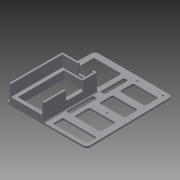
# Autodesk Inventor part: control pod layer a
Saved by Autodesk Inventor 2014 SP1 (Build 180222100, 222)
## iProperties
Created: 2017-06-28
Part Number: control pod layer a
Material: Generic
Document SubType Name: Modeling
Designer: kteo17
Density: 1 g/cm^3
Appearance: Default
Author: kteo17
Autodesk Inventor part; units mm, degrees
ref_plane "YZ Plane" through (0, 0, 0) normal (1, 0, 0) x (0, 1, 0)
ref_plane "XZ Plane" through (0, 0, 0) normal (0, 1, 0) x (-1, 0, 0)
ref_plane "XY Plane" through (0, 0, 0) normal (0, 0, 1) x (1, 0, 0)
sketch "Sketch1" plane through (0, 0, 0) normal (0, 0, 1) x (1, 0, 0)
  line L0 (3.175, 0) -> (146.685, 0)
  line L1 (0, 161.925) -> (149.86, 161.925)
  line L2 (0, 161.925) -> (3.175, 0)
  line L3 (149.86, 161.925) -> (146.685, 0)
  point P0 (0, 0)
  dimension "d60" = 143.51
  dimension "d62" = 161.925
  dimension "d63" = 149.86
  constraints: 8 end point, 1 horizontal
  measures "d60" distance of L0.start L0.end
  measures "d62" distance between parallel lines of L0 L1
  measures "d63" distance of L1.start L1.end
extrude "Extrusion1" add sketch "Sketch1" along normal blind 3.048
fillet "Fillet1" radius 6.35 4 edges at (146.685, 0, 1.524) (149.86, 161.925, 1.524) (0, 161.925, 1.524) (3.175, 0, 1.524)
sketch "Sketch3" plane through (0, 0, 3.048) normal (0, 0, 1) x (1, 0, 0)
  circle A0 centre (59.9281, 7.9375) radius 1.5875
  circle A1 centre (12.7, 7.9375) radius 1.5875
  circle A2 centre (36.3141, 87.9475) radius 1.5875
  point P0 (0, 0)
  dimension "d127" = 3.175
  dimension "d128" = 3.175
  dimension "d129" = 3.175
  dimension "d130" = 47.2281
  dimension "d131" = 80.01
  dimension "d132" = 23.6141
  constraints: 3 centre point
  measures "d127" diameter of A2
  measures "d128" diameter of A1
  measures "d129" diameter of A0
  measures "d130" distance of A0.centre A1.centre
  measures "d131" vertical distance of A1.centre A2.centre
  measures "d132" horizontal distance of A1.centre A2.centre
extrude "Extrusion3" cut sketch "Sketch3" against normal blind 3.048
sketch "Sketch20" plane through (0, 0, 3.048) normal (0, 0, 1) x (1, 0, 0)
  line L0 (79.6253, 161.925) -> (79.6253, 63.5)
  line L1 (79.6253, 63.5) -> (143.6333, 63.5)
  line L2 (143.6333, 63.5) -> (143.6333, 161.925)
  line L3 (82.8003, 161.925) -> (82.8003, 66.675)
  line L4 (82.8003, 66.675) -> (140.4583, 66.675)
  line L5 (140.4583, 66.675) -> (140.4583, 161.925)
  line L6 (143.6333, 161.925) -> (140.4583, 161.925)
  line L7 (82.8003, 161.925) -> (79.6253, 161.925)
  line L8 (143.3843, 161.925) -> (6.4757, 161.925) projected
  point P0 (0, 0)
  dimension "d100" = 98.425
  dimension "d101" = 64.008
  dimension "d102" = 57.658
  dimension "d103" = 95.25
  dimension "d104" = 3.175
  dimension "d105" = 3.175
  constraints: 16 end point, 4 parallel, 2 horizontal, 2 perpendicular, 1 point on line
  measures "d100" distance of L1.end L2.end
  measures "d101" distance of L0.end L1.end
  measures "d102" distance of L3.end L4.end
  measures "d103" distance of L4.end L5.end
  measures "d104" distance between parallel lines of L2 L5
  measures "d105" distance between parallel lines of L3 L0
extrude "Extrusion20" add sketch "Sketch20" along normal blind 31.75 contours L7 L3 L4 L5 L6 L2 L1 L0
sketch "Sketch21" plane through (79.6253, 63.5, 3.048) normal (0, -1, 0) x (1, 0, 0)
  line L0 (6.35, 31.75) -> (31.75, 31.75)
  line L1 (31.75, 31.75) -> (31.75, 13.97)
  line L2 (31.75, 13.97) -> (6.35, 13.97)
  line L3 (6.35, 13.97) -> (6.35, 31.75)
  line L4 (0, 31.75) -> (64.008, 31.75) projected
  point P0 (-79.6253, -3.048)
  dimension "d106" = 25.4
  dimension "d147" = 17.78
  constraints: 8 end point, 2 parallel, 1 horizontal, 1 perpendicular, 1 point on line
  measures "d106" distance of L1.end L2.end
  measures "d147" distance of L0.end L1.end
extrude "Extrusion21" cut sketch "Sketch21" against normal blind 3.175
sketch "Sketch22" plane through (79.6253, 63.5, 3.048) normal (-1, 0, 0) x (0, 0, 1)
  line L0 (31.75, 25.4) -> (17.145, 25.4)
  line L1 (13.97, 28.575) -> (13.97, 53.975)
  line L2 (17.145, 57.15) -> (31.75, 57.15)
  line L3 (31.75, 57.15) -> (31.75, 25.4)
  arc A0 (13.97, 28.575) -> (17.145, 25.4) centre (17.145, 28.575) ccw
  arc A1 (17.145, 57.15) -> (13.97, 53.975) centre (17.145, 53.975) ccw
  line L4 (31.75, 98.425) -> (31.75, 0) projected
  point P0 (-3.048, -63.5)
  dimension "d111" = 3.175
  dimension "d148" = 31.75
  dimension "d149" = 17.78
  constraints: 8 end point, 4 point on circle, 4 tangent, 2 centre point, 2 parallel, 1 equal radius, 1 horizontal, 1 perpendicular, 1 point on line
  measures "d111" radius of A0
  measures "d148" distance between parallel lines of L0 L2
  measures "d149" distance between parallel lines of L1 L3
extrude "Extrusion22" cut sketch "Sketch22" against normal blind 3.175
sketch "Sketch23" plane through (0, 0, 3.048) normal (0, 0, 1) x (1, 0, 0)
  line L0 (140.4583, 66.675) -> (140.4583, 161.925) projected
  line L1 (140.4583, 161.925) -> (82.8003, 161.925) projected
  line L2 (82.8003, 161.925) -> (82.8003, 66.675) projected
  line L3 (82.8003, 66.675) -> (140.4583, 66.675) projected
  line L4 (134.1083, 155.575) -> (89.1503, 155.575)
  line L5 (89.1503, 155.575) -> (89.1503, 69.85)
  line L6 (89.1503, 69.85) -> (134.1083, 69.85)
  line L7 (134.1083, 69.85) -> (134.1083, 155.575)
  point P0 (0, 0)
  dimension "d114" = 44.958
  dimension "d153" = 6.35
  constraints: 8 end point, 2 parallel, 1 horizontal, 1 perpendicular
  measures "d114" distance of L6.end L5.end
  measures "d153" distance between parallel lines of L0 L7
extrude "Extrusion23" add sketch "Sketch23" along normal blind 10.795
sketch "Sketch24" plane through (0, 0, 3.048) normal (0, 0, 1) x (1, 0, 0)
  line L0 (134.1083, 69.85) -> (134.1083, 155.575) projected
  line L1 (134.1083, 155.575) -> (89.1503, 155.575) projected
  line L2 (89.1503, 155.575) -> (89.1503, 69.85) projected
  line L3 (89.1503, 69.85) -> (134.1083, 69.85) projected
  line L4 (89.1503, 55.8893) -> (134.1083, 55.8893)
  line L5 (137.2833, 52.7143) -> (137.2833, 14.2875)
  line L6 (134.1083, 11.1125) -> (89.1503, 11.1125)
  line L7 (85.9753, 14.2875) -> (85.9753, 52.7143)
  arc A0 (89.1503, 55.8893) -> (85.9753, 52.7143) centre (89.1503, 52.7143) ccw
  arc A1 (137.2833, 52.7143) -> (134.1083, 55.8893) centre (134.1083, 52.7143) ccw
  arc A2 (134.1083, 11.1125) -> (137.2833, 14.2875) centre (134.1083, 14.2875) ccw
  arc A3 (85.9753, 14.2875) -> (89.1503, 11.1125) centre (89.1503, 14.2875) ccw
  point P0 (0, 0)
  point P1 (85.9753, 55.8893)
  point P2 (137.2833, 11.1125)
  point P3 (137.2833, 55.8893)
  point P4 (85.9753, 11.1125)
  dimension "d146" = 3.175
  constraints: 8 end point, 8 point on circle, 8 point on line, 8 tangent, 4 centre point, 3 equal radius, 2 parallel, 1 horizontal, 1 perpendicular
  measures "d146" radius of A0
extrude "Extrusion24" cut sketch "Sketch24" against normal blind 3.048
sketch "Sketch25" plane through (0, 0, 3.048) normal (0, 0, 1) x (1, 0, 0)
  line L0 (9.525, 155.575) -> (66.675, 155.575)
  line L1 (69.85, 152.4) -> (69.85, 139.7)
  line L2 (66.675, 136.525) -> (9.525, 136.525)
  line L3 (6.35, 139.7) -> (6.35, 152.4)
  arc A0 (9.525, 155.575) -> (6.35, 152.4) centre (9.525, 152.4) ccw
  arc A1 (6.35, 139.7) -> (9.525, 136.525) centre (9.525, 139.7) ccw
  arc A2 (66.675, 136.525) -> (69.85, 139.7) centre (66.675, 139.7) ccw
  arc A3 (69.85, 152.4) -> (66.675, 155.575) centre (66.675, 152.4) ccw
  line L4 (15.875, 79.375) -> (56.7531, 79.375)
  line L5 (56.7531, 15.875) -> (15.875, 15.875)
  line L6 (15.875, 53.975) -> (56.7531, 53.975)
  line L7 (56.7531, 41.275) -> (15.875, 41.275)
  line L8 (12.7, 19.05) -> (12.7, 38.1)
  line L9 (12.7, 57.15) -> (12.7, 76.2)
  line L10 (59.9281, 76.2) -> (59.9281, 57.15)
  line L11 (59.9281, 38.1) -> (59.9281, 19.05)
  line L12 (15.875, 95.25) -> (58.3406, 95.25)
  line L13 (61.5156, 98.425) -> (61.5156, 120.65)
  line L14 (58.3406, 123.825) -> (15.875, 123.825)
  line L15 (12.7, 120.65) -> (12.7, 98.425)
  line L16 (71.9931, 15.875) -> (73.9103, 15.875)
  line L17 (73.9103, 123.825) -> (71.9931, 123.825)
  arc A4 (15.875, 123.825) -> (12.7, 120.65) centre (15.875, 120.65) ccw
  arc A5 (61.5156, 120.65) -> (58.3406, 123.825) centre (58.3406, 120.65) ccw
  arc A6 (71.9931, 123.825) -> (68.8181, 120.65) centre (71.9931, 120.65) ccw
  arc A7 (77.0853, 120.65) -> (73.9103, 123.825) centre (73.9103, 120.65) ccw
  arc A8 (58.3406, 95.25) -> (61.5156, 98.425) centre (58.3406, 98.425) ccw
  arc A9 (12.7, 98.425) -> (15.875, 95.25) centre (15.875, 98.425) ccw
  arc A10 (15.875, 79.375) -> (12.7, 76.2) centre (15.875, 76.2) ccw
  arc A11 (12.7, 57.15) -> (15.875, 53.975) centre (15.875, 57.15) ccw
  arc A12 (56.7531, 53.975) -> (59.9281, 57.15) centre (56.7531, 57.15) ccw
  arc A13 (59.9281, 76.2) -> (56.7531, 79.375) centre (56.7531, 76.2) ccw
  arc A14 (15.875, 41.275) -> (12.7, 38.1) centre (15.875, 38.1) ccw
  arc A15 (12.7, 19.05) -> (15.875, 15.875) centre (15.875, 19.05) ccw
  arc A16 (59.9281, 38.1) -> (56.7531, 41.275) centre (56.7531, 38.1) ccw
  arc A17 (56.7531, 15.875) -> (59.9281, 19.05) centre (56.7531, 19.05) ccw
  arc A18 (68.8181, 19.05) -> (71.9931, 15.875) centre (71.9931, 19.05) ccw
  arc A19 (73.9103, 15.875) -> (77.0853, 19.05) centre (73.9103, 19.05) ccw
  line L18 (71.9931, 73.025) -> (73.9103, 73.025)
  line L19 (73.9103, 60.325) -> (71.9931, 60.325)
  line L20 (77.0853, 19.05) -> (77.0853, 57.15)
  line L21 (77.0853, 76.2) -> (77.0853, 120.65)
  line L22 (68.8181, 120.65) -> (68.8181, 76.2)
  line L23 (68.8181, 57.15) -> (68.8181, 19.05)
  arc A20 (71.9931, 60.325) -> (68.8181, 57.15) centre (71.9931, 57.15) ccw
  arc A21 (77.0853, 57.15) -> (73.9103, 60.325) centre (73.9103, 57.15) ccw
  arc A22 (68.8181, 76.2) -> (71.9931, 73.025) centre (71.9931, 76.2) ccw
  arc A23 (73.9103, 73.025) -> (77.0853, 76.2) centre (73.9103, 76.2) ccw
  line L24 (85.9753, 14.2875) -> (85.9753, 52.7143) projected
  point P0 (0, 0)
  point P1 (69.85, 136.525)
  point P2 (69.85, 155.575)
  point P3 (6.35, 136.525)
  point P4 (12.7, 79.375)
  point P5 (59.9281, 15.875)
  point P6 (59.9281, 79.375)
  point P7 (12.7, 15.875)
  point P8 (12.7, 53.975)
  point P9 (59.9281, 41.275)
  point P10 (59.9281, 53.975)
  point P11 (12.7, 41.275)
  point P12 (12.7, 95.25)
  point P13 (61.5156, 123.825)
  point P14 (61.5156, 95.25)
  point P15 (12.7, 123.825)
  point P16 (68.8198, 15.875)
  point P17 (77.6872, 123.825)
  point P18 (77.6872, 15.875)
  point P19 (68.8198, 123.825)
  dimension "d133" = 63.5
  dimension "d134" = 19.05
  dimension "d135" = 3.175
  dimension "d152" = 3.175
  dimension "d154" = 3.175
  dimension "d155" = 8.89
  dimension "d156" = 8.89
  constraints: 52 tangent, 48 end point, 48 point on circle, 34 point on line, 24 centre point, 21 equal radius, 16 parallel, 6 horizontal, 6 perpendicular
  measures "d133" distance of point (69.85, 136.525) point (6.35, 136.525)
  measures "d134" distance of point (69.85, 155.575) point (69.85, 136.525)
  measures "d135" radius of A0
  measures "d152" radius of A4
  measures "d154" radius of A20
  measures "d155" distance between parallel lines of L24 L20
  measures "d156" distance between parallel lines of L11 L23
extrude "Extrusion25" cut sketch "Sketch25" against normal blind 3.048
fillet "Fillet8" radius 3.175 2 edges at (79.6253, 112.7125, 3.048) (111.6293, 63.5, 3.048)
sketch "Sketch26" plane through (0, 0, 3.048) normal (0, 0, -1) x (-1, 0, 0)
  arc A0 (-143.3843, 161.925) -> (-143.6333, 161.9201) centre (-143.3843, 155.575) ccw projected
  line L0 (-143.3843, 161.925) -> (-143.6333, 161.925) projected
  line L1 (-143.6333, 161.925) -> (-143.6333, 161.9201) projected
  point P0 (0, 0)
extrude "Extrusion26" cut sketch "Sketch26" against normal blind 50.8
body "Solid1"
